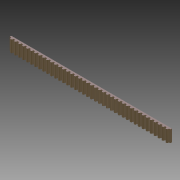
# Autodesk Inventor part: HTD 5M 15mm Riemen
Saved by Autodesk Inventor 2012 SP1 (Build 160190100, 190)
## iProperties
Created: 2013-03-27
Part Number: HTD 5M 15mm Riemen
Material: Default
Document SubType Name: Modeling
Designer: vogel
Density: 1 g/cm^3
Übersetzungsnorm: STEP AP203
Dateiname: C:/Users/Hertelt/Documents/Hochladen/17339900.stp
Postprozessor: Build: 190, Release: 2012 SP1 - Date: Mon 08/08/2011
Gesendete Einheiten: Millimeter
Unbestimmtheit: 1.0000000000000002e-06
Author: vogel
Autodesk Inventor part; units mm, degrees
ref_plane "YZ Plane" through (0, 0, 0) normal (1, 0, 0) x (0, 1, 0)
ref_plane "XZ Plane" through (0, 0, 0) normal (0, 1, 0) x (-1, 0, 0)
ref_plane "XY Plane" through (0, 0, 0) normal (0, 0, 1) x (1, 0, 0)
sketch "Skizze1" plane through (0, 0, 0) normal (0, 0, 1) x (1, 0, 0)
  line L0 (41.4, 8) -> (39.65, 8) projected
  line L1 (39.65, 8) -> (39.65, 7.35) projected
  arc A0 (36.75, 7.35) -> (39.65, 7.35) centre (38.2, 7.35) ccw projected
  line L2 (36.75, 7.35) -> (36.75, 8) projected
  line L3 (36.75, 8) -> (34.65, 8) projected
  line L4 (34.65, 8) -> (34.65, 7.35) projected
  arc A1 (31.75, 7.35) -> (34.65, 7.35) centre (33.2, 7.35) ccw projected
  line L5 (31.75, 7.35) -> (31.75, 8) projected
  line L6 (31.75, 8) -> (29.65, 8) projected
  line L7 (29.65, 8) -> (29.65, 7.35) projected
  arc A2 (26.75, 7.35) -> (29.65, 7.35) centre (28.2, 7.35) ccw projected
  line L8 (26.75, 7.35) -> (26.75, 8) projected
  line L9 (26.75, 8) -> (24.65, 8) projected
  line L10 (24.65, 8) -> (24.65, 7.35) projected
  arc A3 (21.75, 7.35) -> (24.65, 7.35) centre (23.2, 7.35) ccw projected
  line L11 (21.75, 7.35) -> (21.75, 8) projected
  line L12 (21.75, 8) -> (19.65, 8) projected
  line L13 (19.65, 8) -> (19.65, 7.35) projected
  arc A4 (16.75, 7.35) -> (19.65, 7.35) centre (18.2, 7.35) ccw projected
  line L14 (16.75, 7.35) -> (16.75, 8) projected
  line L15 (16.75, 8) -> (14.65, 8) projected
  line L16 (14.65, 8) -> (14.65, 7.35) projected
  arc A5 (11.75, 7.35) -> (14.65, 7.35) centre (13.2, 7.35) ccw projected
  line L17 (11.75, 7.35) -> (11.75, 8) projected
  line L18 (11.75, 8) -> (9.65, 8) projected
  line L19 (9.65, 8) -> (9.65, 7.35) projected
  arc A6 (6.75, 7.35) -> (9.65, 7.35) centre (8.2, 7.35) ccw projected
  line L20 (6.75, 7.35) -> (6.75, 8) projected
  line L21 (6.75, 8) -> (4.65, 8) projected
  line L22 (4.65, 8) -> (4.65, 7.35) projected
  arc A7 (1.75, 7.35) -> (4.65, 7.35) centre (3.2, 7.35) ccw projected
  line L23 (1.75, 7.35) -> (1.75, 8) projected
  line L24 (1.75, 8) -> (0, 8) projected
  line L25 (-8.28, 0) -> (49.68, 0) projected
  line L26 (0, -2) -> (0, 12) projected
  line L27 (0, 10) -> (41.4, 10)
  line L28 (41.4, 10) -> (41.4, 8)
  line L29 (0, 10) -> (0, 8)
  dimension "d0" = 2
  constraints: 6 end point, 2 perpendicular, 1 collinear, 1 point on line
  measures "d0" distance between parallel lines of L27 L24
extrude "Extrusion1" add sketch "Skizze1" along normal blind 15
sketch "Skizze2" plane through (0, 0, -34) normal (0, -1, 0) x (1, 0, 0)
  line L0 (0, 0) -> (41.4, 0) projected
  line L1 (41.4, 34) -> (41.4, 0) projected
  line L2 (0, 34) -> (41.4, 34) projected
  line L3 (0, 34) -> (0, 0) projected
  circle A0 centre (33.2, 6) radius 2.75 projected
  circle A1 centre (8.2, 6) radius 2.75 projected
  circle A2 centre (8.2, 28) radius 2.75 projected
  circle A3 centre (33.2, 28) radius 2.75 projected
extrude "Extrusion2" cut sketch "Skizze2" against normal through all
pattern_linear "Rechteckige Anordnung1" count 5 spacing 40 along (1, 0, 0) of "Extrusion1" first direction both ways yes
